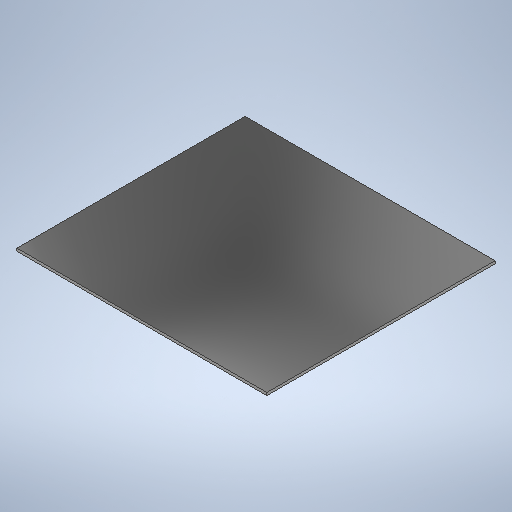
# Autodesk Inventor part: ETROC2 - Simplified
Saved by Autodesk Inventor 2025 (Build 290162000, 162)
## iProperties
Created: 2022-02-01
Part Number: ETROC2 - Simplified
Material: Silicon Nitride
Document SubType Name: Modeling
Designer: Caleb
Density: 3.18 g/cm^3
Appearance: Chrome - Polished Black
Author: Caleb
Autodesk Inventor part; units mm, degrees
ref_plane "YZ Plane" through (0, 0, 0) normal (1, 0, 0) x (0, 1, 0)
ref_plane "XZ Plane" through (0, 0, 0) normal (0, 1, 0) x (-1, 0, 0)
ref_plane "XY Plane" through (0, 0, 0) normal (0, 0, 1) x (1, 0, 0)
sketch "Sketch1" plane through (0, 0, 0) normal (0, 1, 0) x (-1, 0, 0)
  point P0 (0, 0)
sketch "Sketch2" plane through (0, 0, 0) normal (0, 1, 0) x (-1, 0, 0)
  line L0 (-11.5, 10.5) -> (11.5, 10.5)
  line L1 (11.5, 10.5) -> (11.5, -10.5)
  line L2 (11.5, -10.5) -> (-11.5, -10.5)
  line L3 (-11.5, -10.5) -> (-11.5, 10.5)
  line L4 (-11.5, 10.5) -> (11.5, -10.5) construction
  line L5 (11.5, 10.5) -> (-11.5, -10.5) construction
  point P0 (0, 0)
  dimension "d0" = 21
  dimension "d1" = 23
  constraints: 12 end point, 2 midpoint, 2 parallel, 1 horizontal, 1 perpendicular
  measures "d0" distance of L0.end L1.end
  measures "d1" distance of L0.start L0.end
extrude "Extrusion1" add sketch "Sketch2" along normal blind 0.25
body "Solid1"
